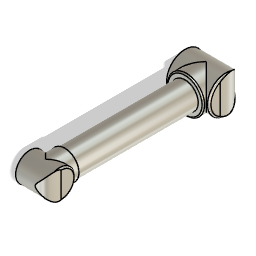
Link3 v17 (Autodesk Fusion 360 design; units mm, degrees)
Autodesk Fusion 360 part; units mm, degrees
sketch "Boceto1" plane through (0, 0, 0) normal (0, 0, 1) x (1, 0, 0)
  circle A0 centre (0, 0) radius 75
  dimension "d1" = 150
  constraint coincident A0.centre origin
  measures "d1" diameter of A0
extrude "Extruir1" add sketch "Boceto1" along normal blind 173.5
sketch "Boceto2" plane through (0, 0, 0) normal (1, 0, 0) x (0, 0, -1)
  circle A0 centre (-86.75, 0) radius 75
  line L0 (-173.5, 75) -> (-173.5, -75)
  dimension "d4" = 150
  dimension "d5" = 86.75
  measures "d4" diameter of A0
  measures "d5" distance of A0.centre L0
extrude "Extruir2" add sketch "Boceto2" along normal blind 87
sketch "Boceto3" plane through (87, 0, 0) normal (1, 0, 0) x (0, 0, -1)
  circle A0 centre (-86.75, 0) radius 75
  circle A1 centre (-86.75, 0) radius 54.25
  circle A2 centre (-86.75, 0) radius 39.25
  dimension "d8" = 108.5
  dimension "d30" = 78.5
  constraint concentric A0 A1
  constraint concentric A0 A2
  measures "d8" diameter of A1
  measures "d30" diameter of A2
extrude "Extruir3" add sketch "Boceto3" along normal blind 490.5 contours A1 | A2
sketch "Boceto4" plane through (577.5, 0, 0) normal (1, 0, 0) x (0, 0, -1)
  circle A0 centre (-86.75, 0) radius 54.25
  circle A1 centre (-86.75, 0) radius 58
  dimension "d11" = 116
  constraint concentric A0 A1
  measures "d11" diameter of A1
extrude "Extruir4" add sketch "Boceto4" along normal blind 78.5 contours A0 | A1
sketch "Boceto6" plane through (0, 0, 0) normal (0, 0, 1) x (1, 0, 0)
ref_plane "PlanoDeObra1" through (656, 0, 144.75) normal (0, 0, 1) x (1, 0, 0)
ref_plane "PlanoDeObra2" through (0, 0, 86.75) normal (0, 0, 1) x (1, 0, 0)
sketch "Boceto8" plane through (0, 0, 86.75) normal (0, 0, 1) x (1, 0, 0)
  circle A0 centre (656, 0) radius 58
  line L0 (577.5, -58) -> (577.5, 58)
  dimension "d18" = 116
  dimension "d19" = 78.5
  measures "d18" diameter of A0
  measures "d19" distance of A0.centre L0
extrude "Extruir5" add sketch "Boceto8" along normal mid plane 128.5
fillet "Empalme1" radius 7 1 edges at (-69.9246, -27.1212, 0)
fillet "Empalme2" radius 5 1 edges at (87, -27.1212, 156.6746)
fillet "Empalme3" radius 6 1 edges at (601.925, 20.9737, 22.5)
sketch "Sketch9" plane through (0, 0, 0) normal (0, 1, 0) x (1, 0, 0)
  spline S0 degree 5 poles (30, 0) (20.6021, 0) (3.1379, -0.6783) (-19.0662, -3.7294) (-41.6367, -11.562) (-60.9649, -27.3594) (-70.479, -45.6365) (-74.1777, -63.4911) (-75, -77.4821) (-75, -85) knots 0 0 0 0 0 0 0.2 0.4 0.6 0.8 1 1 1 1 1 1
  line L0 (-75, -70) -> (-75, -100)
  line L1 (50, 0) -> (10, 0)
  line L2 (-75, -85) -> (-75, 0)
  line L3 (-75, 0) -> (30, 0)
  constraint midpoint S0.end L0
  constraint midpoint S0.start L1
  constraint perpendicular L0 L3
extrude "Extrude6" cut sketch "Sketch9" along normal through all and the other way through all
sketch "Sketch10" plane through (0, 0, 0) normal (0, 1, 0) x (1, 0, 0)
  spline S0 degree 5 poles (625, -20) (630.4011, -20) (641.0532, -20.3288) (656.5809, -21.8079) (676.1994, -25.8618) (697.3361, -35.9404) (709.3735, -50.4365) (714.1562, -66.716) (715.1454, -80.3545) (715.0898, -87.8708) knots 0 0 0 0 0 0 0.2 0.4 0.6 0.8 1 1 1 1 1 1
  line L0 (715.1841, -75.1292) -> (714.9954, -100.6125)
  line L1 (615, -20) -> (635, -20)
  line L2 (625, -20) -> (715, -20)
  line L3 (715, -20) -> (715.0898, -87.8708)
  constraint midpoint S0.end L0
  constraint midpoint S0.start L1
  constraint horizontal L2
extrude "Extrude7" cut sketch "Sketch10" along normal through all and the other way through all contours S0 L1 L2 L3
extrude "Extrude8" cut sketch "Boceto3" along normal blind 490.5 contours A2
move_body "Desplazar1" bodies 1 to x (0, 1, 0) y (0, 0, 1) z (1, 0, 0) at (0.25, -87, 86.75)
move_body "Desplazar2" bodies 1 to x (1, 0, 0) y (0, 1, 0) z (0, 0, 1) at (-100, 100, -100)
move_body "Desplazar3" bodies 1 to x (0, -1, 0) y (1, 0, 0) z (0, 0, 1) at (182.25, 720.25, 700)
move_body "Desplazar4" bodies 1 to x (1, 0, 0) y (0, 1, 0) z (0, 0, 1) at (-120, 0, 30)
move_body "Desplazar5" bodies 1 to x (1, 0, 0) y (0, 1, 0) z (0, 0, 1) at (-75, -646.5, -716.5)
sketch "Sketch11" plane through (0, 0, 0) normal (0, 1, 0) x (1, 0, 0)
sketch "Sketch12" plane through (0, 0, 0) normal (0, 0, 1) x (1, 0, 0)
  line L0 (650, 22.5) -> (650, 0)
  dimension "d36" = 22.5
  constraint vertical L0
  measures "d36" distance of L0.start L0.end
sketch "Sketch13" plane through (0, 22.5, 0) normal (0, -1, 0) x (1, 0, 0)
  circle A0 centre (656.25, 0.25) radius 58
  line L0 (0, 0) -> (656.25, 0.25)
  dimension "d37" = 656.25
  constraint coincident L0.start origin
  constraint coincident A0.centre L0.end
  measures "d37" horizontal distance of L0.start A0.centre
sketch "Sketch14" plane through (0, 0, 0) normal (0, 0, 1) x (1, 0, 0)
  line L0 (90.9, 141) -> (90.9, 32.5)
  line L1 (90.9, 32.5) -> (90.9, 0)
  dimension "d38" = 32.5
  dimension "d39" = 108.5
  constraint vertical L0
  constraint vertical L1
  measures "d38" distance of L0.end L1.end
  measures "d39" distance of L0.start L0.end
